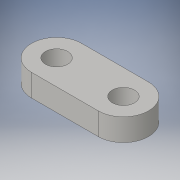
# Autodesk Inventor part: A8-0015
Saved by Autodesk Inventor 2016 SP2 (Build 200236200, 236)
## iProperties
Created: 2017-04-22
Part Number: A8-0015
Material: Generic
Document SubType Name: Modeling
Designer: EV
Density: 1 g/cm^3
Appearance: Default
Author: EV
Autodesk Inventor part; units mm, degrees
ref_plane "YZ Plane" through (0, 0, 0) normal (1, 0, 0) x (0, 1, 0)
ref_plane "XZ Plane" through (0, 0, 0) normal (0, 1, 0) x (-1, 0, 0)
ref_plane "XY Plane" through (0, 0, 0) normal (0, 0, 1) x (1, 0, 0)
sketch "Sketch1" plane through (0, 0, 0) normal (0, 1, 0) x (-1, 0, 0)
  line L0 (0, 0) -> (-21, 0) construction
  line L1 (-4.5, 4.5) -> (-16.5, 4.5)
  line L2 (-16.5, -4.5) -> (-4.5, -4.5)
  arc A0 (-4.5, -4.5) -> (-4.5, 4.5) centre (-4.5, 0) ccw
  arc A1 (-16.5, 4.5) -> (-16.5, -4.5) centre (-16.5, 0) ccw
  point P0 (-10.5, 0)
  dimension "d0" = 9
  dimension "d1" = 21
  constraints: 8 end point, 6 point on circle, 4 tangent, 2 centre point, 2 point on line, 1 horizontal, 1 midpoint, 1 parallel
  measures "d0" distance between parallel lines of L2 L1
  measures "d1" distance of L0.start L0.end
extrude "Extrusion1" add sketch "Sketch1" along normal blind 4
hole "Hole1" at (4.5, 4, 0) direction (0, -1, 0) diameter 4 end through all
hole "Hole2" at (16.5, 4, 0) direction (0, -1, 0) diameter 4 end through all
body "Solid1"
